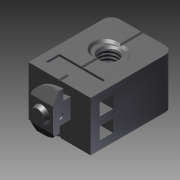
# Autodesk Inventor part: HCBR5
Saved by Autodesk Inventor 2015 SP1 (Build 190203100, 203)
## iProperties
Category: Hardware
Company: MISUMI
Created: 2015-01-26
Part Number: HCBR5
Catalog Web Link: http://us.misumi-ec.com/vona2/detail/110302262610/
Description: HCBR, HCBRB-Panel Support Brackets - Resin Type - for Center Mounting (One-Touch Mounting)
Vendor: MISUMI
Document SubType Name: Modeling
Designer: PARTuser1
Manufacturer: MISUMI
Mass: 3.24843 g
Surface Area: 20.515 cm^2
Volume: 3.24843 cm^3
Density: 1 g/cm^3
Material: Generic
Appearance: PSOLRGB-191-191-191
Stock Number: HCBRB5
PSOL_IDENT_0: {\\10.0.0.236\data_v8\23d-libs\misumi\metric\39_accessories_for_al_extrusions\hcbr.prj},162 {VTYP=3D
PSOL_IDENT_1: },{NB=HCBR5},{LINA=HCBR5},{NN=HCBR, HCBRB},{DATE=17.11.2014 05:30:47},{GEOMDATE=19.05.2009 09:26:00}
PSOL_IDENT_2: ,{VERSION=},{LINEID=10},{LINESUBID=-1},{WBVAR=COLOR}  {NB=HCBR5},{LINA=HCBR5},{KT=DUMMY},{PN=HCBR5},
PSOL_IDENT_3: {COLOR=},{TS=HCBR},{MAT=Polyamide},{NO=5},{MASS=4.3},{A=12},{DIFF=3 or 5},{COL=0.75,0.75,0.75,0.00},
PSOL_IDENT_4: {M=5},{KDM=4.134}
SUPPLIER: MISUMI
ARTICLENO: HCBR5
BOMINFO: HCBR5
CREATOR: CADENAS GmbH
Title: Panel Mount
Author: Misumi
Autodesk Inventor part; units mm, degrees
ref_plane "YZ Plane" through (0, 0, 0) normal (1, 0, 0) x (0, 1, 0)
ref_plane "XZ Plane" through (0, 0, 0) normal (0, 1, 0) x (-1, 0, 0)
ref_plane "XY Plane" through (0, 0, 0) normal (0, 0, 1) x (1, 0, 0)
sketch "Sketch_1" plane through (0, 0, 0) normal (0, 0, 1) x (1, 0, 0)
  line L0 (0, 22) -> (0, 4)
  line L1 (0, 4) -> (15, 4)
  line L2 (15, 4) -> (15, 22)
  arc A0 (15, 22) -> (13, 24) centre (13, 22) ccw
  line L3 (13, 24) -> (2, 24)
  arc A1 (2, 24) -> (0, 22) centre (2, 22) ccw
  constraints: 8 end point, 4 point on circle, 2 centre point
extrude "Extrusion1" add sketch "Sketch_1" against normal blind 12
sketch "Sketch_8" plane through (6.5, 0, 0) normal (1, 0, 0) x (0, 0, -1)
  line L0 (0, 16) -> (12, 16)
  line L1 (12, 16) -> (12, 13)
  line L2 (12, 13) -> (11.5, 13.5)
  line L3 (11.5, 13.5) -> (0.5, 13.5)
  line L4 (0.5, 13.5) -> (0, 13)
  line L5 (0, 13) -> (0, 16)
  line L6 (0, 16) -> (12, 16)
  constraints: 14 end point
revolve "Revolution1" cut sketch "Sketch_8" angle 360 about axis through (6.5, 16, 0) along (0, 0, 1)
sketch "Sketch_9" plane through (8.5, 0, 0) normal (1, 0, 0) x (0, 0, -1)
  line L0 (0, 16) -> (12, 16)
  line L1 (12, 16) -> (12, 13)
  line L2 (12, 13) -> (11.5, 13.5)
  line L3 (11.5, 13.5) -> (0.5, 13.5)
  line L4 (0.5, 13.5) -> (0, 13)
  line L5 (0, 13) -> (0, 16)
  line L6 (0, 16) -> (12, 16)
  constraints: 14 end point
revolve "Revolution2" cut sketch "Sketch_9" angle 360 about axis through (8.5, 16, 0) along (0, 0, 1)
sketch "Sketch_10" plane through (6.5, 0, 0) normal (1, 0, 0) x (0, 0, -1)
  line L0 (0, 13) -> (0.5, 13.5)
  line L1 (0.5, 13.5) -> (11.5, 13.5)
  line L2 (11.5, 13.5) -> (12, 13)
  line L3 (12, 13) -> (12, 19)
  line L4 (12, 19) -> (11.5, 18.5)
  line L5 (11.5, 18.5) -> (0.5, 18.5)
  line L6 (0.5, 18.5) -> (0, 19)
  line L7 (0, 19) -> (0, 13)
  constraints: 16 end point
extrude "Extrusion2" cut sketch "Sketch_10" along normal blind 2
sketch "Sketch_7" plane through (7.5, 0, 0) normal (1, 0, 0) x (0, 0, -1)
  line L0 (-0.5, 1.15) -> (2.1, -0.3)
  line L1 (2.1, -0.3) -> (7.9, -0.3)
  line L2 (7.9, -0.3) -> (10.5, 1.15)
  line L3 (10.5, 1.15) -> (10.5, 2.5)
  line L4 (10.5, 2.5) -> (7.9, 2.5)
  line L5 (7.9, 2.5) -> (7.9, 4)
  line L6 (7.9, 4) -> (2.1, 4)
  line L7 (2.1, 4) -> (2.1, 2.5)
  line L8 (2.1, 2.5) -> (-0.5, 2.5)
  line L9 (-0.5, 2.5) -> (-0.5, 1.15)
  constraints: 20 end point
sketch "Sketch_3" plane through (0, 0, 0) normal (1, 0, 0) x (0, 1, 0)
  line L0 (6.2, -2) -> (6.2, -5)
  line L1 (6.2, -5) -> (9.45, -5)
  line L2 (9.45, -5) -> (9.45, -2)
  line L3 (9.45, -2) -> (6.2, -2)
  constraints: 8 end point
sketch "Sketch_5" plane through (0, 0, 0) normal (1, 0, 0) x (0, 1, 0)
  line L0 (6.2, -7) -> (6.2, -10)
  line L1 (6.2, -10) -> (9.45, -10)
  line L2 (9.45, -10) -> (9.45, -7)
  line L3 (9.45, -7) -> (6.2, -7)
  constraints: 8 end point
extrude "Extrusion3" cut sketch "Sketch_3" along normal blind 15
extrude "Extrusion4" cut sketch "Sketch_5" along normal blind 15
sketch "Sketch_6" plane through (0, 0, 0) normal (0, 0, 1) x (1, 0, 0)
  line L0 (2, 6.2) -> (13, 6.2)
  line L1 (13, 6.2) -> (13, 9.45)
  line L2 (13, 9.45) -> (2, 9.45)
  line L3 (2, 9.45) -> (2, 6.2)
  constraints: 8 end point
extrude "Extrusion5" cut sketch "Sketch_6" against normal blind 0.5
sketch "Sketch_11" plane through (0, 0, 0) normal (0, 1, 0) x (-1, 0, 0)
  line L0 (-7.2, 0) -> (-7.8, 0)
  line L1 (-7.8, 0) -> (-7.5, -0.3)
  line L2 (-7.5, -0.3) -> (-7.2, 0)
  constraints: 6 end point
extrude "Extrusion6" cut sketch "Sketch_11" along normal blind 25
sketch "Sketch_12" plane through (0, 0, 0) normal (0, 1, 0) x (-1, 0, 0)
  line L0 (-7.2, -12) -> (-7.5, -11.7)
  line L1 (-7.5, -11.7) -> (-7.8, -12)
  line L2 (-7.8, -12) -> (-7.2, -12)
  constraints: 6 end point
extrude "Extrusion7" cut sketch "Sketch_12" along normal blind 25
extrude "Extrusion8" add sketch "Sketch_7" along normal mid plane 5.4
sketch "Sketch_2" plane through (7.5, 0, 0) normal (1, 0, 0) x (0, 0, -1)
  line L0 (5, -0.3) -> (5, -1.3)
  line L1 (5, -1.3) -> (3.364, -1.3)
  line L2 (3.364, -1.3) -> (3, -0.3)
  line L3 (3, -0.3) -> (5, -0.3)
  line L4 (5, -0.3) -> (5, -1.3)
  constraints: 10 end point
revolve "Revolution3" add sketch "Sketch_2" angle 360 about axis through (7.5, -0.3, -5) along (0, 1, 0)
sketch "Sketch_4" plane through (0, 0, 0) normal (0, 1, 0) x (-1, 0, 0)
  line L0 (-3.8, 1.5) -> (-10.2, 1.5)
  line L1 (-10.2, 1.5) -> (-10.2, 0.5)
  line L2 (-10.2, 0.5) -> (-8.7, 0.5)
  arc A0 (-4.8, -1.5) -> (-8.7, 0.5) centre (-8.8008, -4.499) ccw
  line L3 (-4.8, -1.5) -> (-3.8, -1.5)
  line L4 (-3.8, -1.5) -> (-3.8, 1.5)
  constraints: 10 end point, 2 point on circle, 1 centre point
extrude "Extrusion9" cut sketch "Sketch_4" along normal blind 3
sketch "Sketch_13" plane through (0, 0, 0) normal (0, 1, 0) x (-1, 0, 0)
  line L0 (-4.8, -10.5) -> (-6.3, -10.5)
  arc A0 (-10.2, -8.5) -> (-6.3, -10.5) centre (-6.1992, -5.501) ccw
  line L1 (-10.2, -8.5) -> (-11.2, -8.5)
  line L2 (-11.2, -8.5) -> (-11.2, -11.5)
  line L3 (-11.2, -11.5) -> (-4.8, -11.5)
  line L4 (-4.8, -11.5) -> (-4.8, -10.5)
  constraints: 10 end point, 2 point on circle, 1 centre point
extrude "Extrusion10" cut sketch "Sketch_13" along normal blind 3
sketch "Sketch_14" plane through (10.2, 0, 0) normal (1, 0, 0) x (0, 0, -1)
  circle A0 centre (5, 1.5) radius 0.7
  constraints: 1 centre point
extrude "Extrusion11" cut sketch "Sketch_14" against normal blind 0.3
sketch "Sketch_15" plane through (0, 0, -0.5) normal (0, 0, 1) x (1, 0, 0)
  arc A0 (6.5, 18.5) -> (6.5, 13.5) centre (6.5, 16) ccw
  line L0 (6.5, 13.5) -> (8.5, 13.5)
  arc A1 (8.5, 13.5) -> (8.5, 18.5) centre (8.5, 16) ccw
  line L1 (8.5, 18.5) -> (6.5, 18.5)
  constraints: 4 end point, 4 point on circle, 2 centre point
extrude "Extrusion12" add sketch "Sketch_15" against normal blind 11
sketch "Sketch_16" plane through (7.5, 0, 0) normal (1, 0, 0) x (0, 0, -1)
  line L0 (0.5, 16) -> (11.5, 16)
  line L1 (11.5, 16) -> (11.5, 13.5)
  line L2 (11.5, 13.5) -> (11.067, 13.933)
  line L3 (11.067, 13.933) -> (0.933, 13.933)
  line L4 (0.933, 13.933) -> (0.5, 13.5)
  line L5 (0.5, 13.5) -> (0.5, 16)
  line L6 (0.5, 16) -> (11.5, 16)
  constraints: 14 end point
revolve "Revolution4" cut sketch "Sketch_16" angle 360 about axis through (7.5, 16, -0.5) along (0, 0, 1)
thread "Thread1" size "M5x0.8" class "6H" standard "ISO Metric profile" full length
sketch "Sketch_17" plane through (0, 4, 0) normal (0, 1, 0) x (1, 0, 0)
  line L0 (2, 10) -> (2, 0)
  line L1 (2, 0) -> (12, 0)
  line L2 (12, 0) -> (12, 10)
  line L3 (12, 10) -> (2, 10)
  line L4 (4.8, 3.0522) -> (10.2, 2.1)
  line L5 (10.2, 2.1) -> (10.2, 6.9478)
  line L6 (10.2, 6.9478) -> (4.8, 7.9)
  line L7 (4.8, 7.9) -> (4.8, 3.0522)
  constraints: 16 end point
extrude "Extrusion13" cut sketch "Sketch_17" against normal blind 1.5
sketch "Sketch_18" plane through (0, 2.5, 0) normal (0, 1, 0) x (1, 0, 0)
  line L0 (11.7, 15) -> (11.7, -5)
  line L1 (2.8, 3.4048) -> (2.8, -5)
  line L2 (2.8, -5) -> (11.2, -5)
  line L3 (11.2, -5) -> (11.2, 1.9237)
  line L4 (11.2, 1.9237) -> (2.8, 3.4048)
  constraints: 10 end point
revolve "Revolution5" cut sketch "Sketch_18" angle 10 about axis through (11.7, 2.5, -15) along (0, 0, 1)
sketch "Sketch_19" plane through (0, 2.5, 0) normal (0, 1, 0) x (1, 0, 0)
  line L0 (3.3, -5) -> (3.3, 15)
  line L1 (3.8, 8.0763) -> (12.2, 6.5952)
  line L2 (12.2, 6.5952) -> (12.2, 15)
  line L3 (12.2, 15) -> (3.8, 15)
  line L4 (3.8, 15) -> (3.8, 8.0763)
  constraints: 10 end point
revolve "Revolution6" cut sketch "Sketch_19" angle 10 about axis through (3.3, 2.5, 5) along (0, 0, -1)
body "Solid1"
